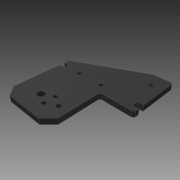
# Autodesk Inventor part: z_axis_top
Saved by Autodesk Inventor 2014 (Build 180170000, 170)
## iProperties
Created: 2013-12-06
Part Number: z_axis_top
Material: Generic
Document SubType Name: Modeling
Designer: buben
Density: 1 g/cm^3
Appearance: Anodized - Dark Gray
Author: buben
Subject: Laser Cutted
Autodesk Inventor part; units mm, degrees
ref_plane "YZ Plane" through (0, 0, 0) normal (1, 0, 0) x (0, 1, 0)
ref_plane "XZ Plane" through (0, 0, 0) normal (0, 1, 0) x (-1, 0, 0)
ref_plane "XY Plane" through (0, 0, 0) normal (0, 0, 1) x (1, 0, 0)
sketch "Sketch1" plane through (0, 0, 0) normal (0, 0, 1) x (1, 0, 0)
  line L0 (0, 0) -> (0, -52)
  line L1 (0, -52) -> (10, -62)
  line L2 (10, -62) -> (50, -62)
  line L3 (50, -62) -> (60, -52)
  line L4 (60, -52) -> (60, -6)
  line L5 (0, 0) -> (6, 0)
  line L6 (6, 0) -> (6, 6)
  line L7 (6, 6) -> (0, 6)
  line L8 (0, 6) -> (0, 12)
  line L9 (0, 12) -> (76, 50)
  line L10 (60, -6) -> (96, -6)
  line L11 (96, -6) -> (96, 0)
  line L12 (96, 0) -> (90, 0)
  line L13 (90, 0) -> (90, 6)
  line L14 (90, 6) -> (96, 6)
  line L15 (96, 6) -> (96, 50)
  line L16 (96, 50) -> (76, 50)
  circle A0 centre (49, -42) radius 2.5
  circle A1 centre (26, -42) radius 4
  dimension "d0" = 45
  dimension "d1" = 10
  dimension "d2" = 8
  dimension "d3" = 5
  dimension "d4" = 23
  dimension "d5" = 6
  dimension "d6" = 6
  dimension "d7" = 6
  dimension "d8" = 42
  dimension "d9" = 6
  dimension "d10" = 26
  dimension "d11" = 44
  dimension "d12" = 20
  dimension "d14" = 6
  dimension "d15" = 84
  dimension "d16" = 60
  dimension "d17" = 20
  constraints: 34 end point, 7 parallel, 5 collinear, 5 perpendicular, 2 centre point, 2 horizontal alignment, 1 vertical
  measures "d0" angle of L0 L1
  measures "d1" horizontal distance of L1.end L0.end
  measures "d2" diameter of A1
  measures "d3" diameter of A0
  measures "d4" distance of A1.centre A0.centre
  measures "d5" distance of L5.end L6.end
  measures "d6" distance of L0.start L5.end
  measures "d7" distance of L13.end L14.end
  measures "d8" distance from line of A1.centre L5
  measures "d9" distance of L10.end L11.end
  measures "d10" distance from line of A1.centre L0
  measures "d11" distance of L14.end L15.end
  measures "d12" distance of L15.end L9.end
  measures "d14" distance of L7.end L8.end
  measures "d15" distance between parallel lines of L13 L6
  measures "d16" distance between parallel lines of L4 L0
  measures "d17" distance from line of L2 A1.centre
extrude "Extrusion1" add sketch "Sketch1" along normal blind 6
sketch "Sketch16" plane through (0, 0, 6) normal (0, 0, 1) x (1, 0, 0)
  circle A0 centre (26, -42) radius 4 projected
  circle A1 centre (49, -42) radius 2.5 projected
  line L0 (6, 0) -> (0, 0) projected
  circle A2 centre (37.5, -36) radius 2.25
  circle A3 centre (37.5, -48) radius 2.25
  line L1 (37.5, -36) -> (37.5, -48) construction
  line L2 (26, -42) -> (49, -42) construction
  point P0 (37.5, -42)
  dimension "d119" = 4.5
  dimension "d120" = 12
  constraints: 4 end point, 2 centre point, 2 midpoint, 2 perpendicular, 1 equal radius, 1 vertical alignment
  measures "d119" diameter of A3
  measures "d120" distance of L1.start L1.end
extrude "Extrusion13" cut sketch "Sketch16" against normal through all contours A2 | A3
chamfer "Chamfer5" distance 2 angle 45 3 edges at (60, -6, 3) (96, -6, 3) (96, 50, 3)
sketch "Sketch22" plane through (0, 0, 6) normal (0, 0, 1) x (1, 0, 0)
  line L0 (6, 6) -> (6, 0) projected
  line L1 (0, 0) -> (0, -52) projected
  circle A0 centre (25, 3) radius 2.25
  circle A1 centre (52.551, 3) radius 2.25
  point P0 (6, 3)
  dimension "d165" = 25
  dimension "d166" = 4.5
  dimension "d167" = 4.5
  dimension "d168" = 27.551
  constraints: 2 centre point, 2 horizontal alignment, 1 midpoint
  measures "d165" distance from line of L1 A0.centre
  measures "d166" diameter of A0
  measures "d167" diameter of A1
  measures "d168" distance of A0.centre A1.centre
extrude "Extrusion19" cut sketch "Sketch22" against normal through all
sketch "Sketch23" plane through (0, 0, 6) normal (0, 0, 1) x (1, 0, 0)
  line L0 (90, 6) -> (96, 6) projected
  line L1 (96, 6) -> (96, 48) projected
  circle A0 centre (84, 33.731) radius 2.25
  dimension "d171" = 27.731
  dimension "d172" = 4.5
  dimension "d173" = 12
  constraints: 1 centre point
  measures "d171" distance from line of L0 A0.centre
  measures "d172" diameter of A0
  measures "d173" distance from line of L1 A0.centre
extrude "Extrusion20" cut sketch "Sketch23" against normal through all
body "Solid1"
